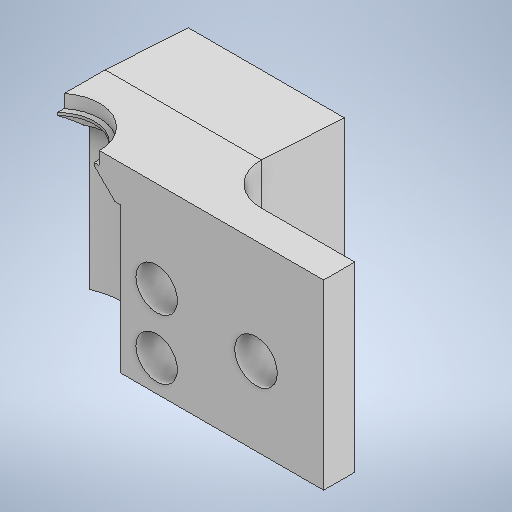
# Autodesk Inventor part: JH_int_Greiferkoerper_Gegenstueck
Saved by Autodesk Inventor 2025.1 (Build 291241000, 241)
## iProperties
Created: 2025-06-16
Part Number: JH_int_Greiferkoerper_Gegenstueck
Material: Generisch
Document SubType Name: Modeling
Designer: Jakob
Density: 1 g/cm^3
Appearance: Vorgabe
Author: Jakob
Autodesk Inventor part; units mm, degrees
ref_plane "YZ Plane" through (0, 0, 0) normal (1, 0, 0) x (0, 1, 0)
ref_plane "XZ Plane" through (0, 0, 0) normal (0, 1, 0) x (-1, 0, 0)
sketch "Skizze1" plane through (0, 0, 0) normal (0, 0, 1) x (1, 0, 0)
  line L0 (6.45, 0) -> (15, 0)
  line L1 (15, 0) -> (15, 15)
  line L2 (15, 15) -> (0, 15)
  line L3 (0, 15) -> (0, 3.0582)
  arc A0 (6.45, 0) -> (0, 3.0582) centre (2.5, 0) ccw
  line L4 (-3, 0) -> (18, 0) projected
  line L5 (0, -3) -> (0, 18) projected
  point P0 (0, 0)
  dimension "d0" = 15
  dimension "d1" = 15
  dimension "d2" = 7.9
  dimension "d3" = 2.5
  constraints: 8 end point, 2 parallel, 2 point on circle, 2 point on line, 1 centre point, 1 collinear, 1 horizontal, 1 perpendicular
  measures "d0" distance of L0.end L1.end
  measures "d1" distance of L1.end L2.end
  measures "d2" diameter of A0
  measures "d3" distance from line of L3 A0.centre
extrude "Extrusion1" add sketch "Skizze1" along normal mid plane 17.5 contours A0 L3 L2 L1 L0
ref_plane "Arbeitsebene1" through (0, 0, 7.5) normal (0, 0, 1) x (1, 0, 0)
sketch "Skizze2" plane through (0, 0, 7.5) normal (0, 0, 1) x (1, 0, 0)
  circle A0 centre (2.5, 0) radius 3.95
  arc A1 (6.45, 0) -> (0, 3.0582) centre (2.5, 0) ccw projected
  circle A2 centre (2.5, 0) radius 3.45
  line L0 (0, 3.0582) -> (0, 2.3775)
  line L1 (15, 0) -> (6.45, 0) projected
  line L2 (6.45, 0) -> (5.95, 0)
  point P0 (0, 0)
  point P1 (0, 3.0582)
  dimension "d7" = 7.9
  dimension "d8" = 6.9
  constraints: 4 end point, 2 centre point, 2 point on circle, 1 coincident, 1 collinear, 1 concentric, 1 vertical
  measures "d7" diameter of A0
  measures "d8" diameter of A2
extrude "Extrusion2" add sketch "Skizze2" against normal up to surface (16.25 mm away) contours L2 A2 L0 A0 picked at (6.25, 0.2945)
sketch "Skizze4" plane through (15, 0, 8.75) normal (1, 0, 0) x (0, 0, -1)
  line L0 (17.5, 3) -> (0, 3)
  line L1 (0, 3) -> (0, 0)
  line L2 (0, 0) -> (17.5, 0)
  line L3 (17.5, 0) -> (17.5, 3)
  line L4 (17.5, 15) -> (17.5, 0) projected
  line L5 (0, 0) -> (0, 15) projected
  line L6 (17.5, 0) -> (0, 0) projected
  point P0 (8.75, 0)
  dimension "d11" = 3
  constraints: 8 end point, 3 collinear, 2 parallel, 1 horizontal, 1 perpendicular
  measures "d11" distance between parallel lines of L2 L0
extrude "Extrusion3" add sketch "Skizze4" along normal blind 13
fillet "Rundung1" radius 4 1 edges at (15, 3, 0)
sketch "Skizze5" plane through (28, 3, 8.75) normal (0, 1, 0) x (1, 0, 0)
  line L0 (-9, 0) -> (0, 0) projected
  line L1 (0, 17.5) -> (0, 0) projected
  point P0 (-28, 8.75)
  point P1 (-6.5, 10)
  dimension "d15" = 10
  dimension "d16" = 6.5
  measures "d15" distance from line of L0 point (-6.5, 10)
  measures "d16" distance from line of L1 point (-6.5, 10)
hole "Bohrung1" at (21.5, 3, -1.25) direction (0, -1, 0) diameter 4.1 end through all
sketch "Skizze6" plane through (5.95, 0, -8.75) normal (0, -1, 0) x (1, 0, 0)
  line L0 (0, 0) -> (22.05, 0) projected
  line L1 (-11.55, 8.75) -> (27.65, 8.75) projected
  line L2 (0, 16.25) -> (0, 0) projected
  point P0 (-5.95, 8.75)
  point P1 (6, 3)
  point P2 (6, 8.75)
  dimension "d24" = 3
  dimension "d25" = 6
  constraints: 1 point on line, 1 vertical alignment
  measures "d24" distance from line of L0 point (6, 3)
  measures "d25" distance from line of L2 point (6, 3)
hole "Bohrung2" at (11.95, 0, -5.75) at (11.95, 0, 0) direction (0, 1, 0) diameter 4 depth 8 tip angle 118
sketch "Skizze7" plane through (0, 0, -8.75) normal (0, 0, -1) x (-1, 0, 0)
  circle A0 centre (-2.5, 0) radius 6
  arc A1 (0, 2.3775) -> (-5.95, 0) centre (-2.5, 0) ccw projected
  line L0 (-5.95, 0) -> (-8.5, 0)
  line L1 (-5.95, 0) -> (-28, 0) projected
  line L2 (0, 2.3775) -> (0, 15) projected
  line L3 (0, 2.3775) -> (0, 5.4544)
  point P0 (0, 0)
  dimension "d34" = 12
  constraints: 4 end point, 2 point on circle, 2 point on line, 1 centre point, 1 concentric
  measures "d34" diameter of A0
extrude "Extrusion4" cut sketch "Skizze7" against normal blind 14 contours L2 A1 L0 A0 picked at (-7.6008, 0.4409)
chamfer "Fasen1" distance 2 angle 45 1 edges at (3.7801, 3.2037, 5.25)
sketch "Skizze8" plane through (0, 3.0582, 8.75) normal (-1, 0, 0) x (0, 0, 1)
  line L0 (0, 3.9418) -> (0, 11.9418) projected
  line L1 (0, 3.9418) -> (-0.5, 11.9418)
  line L2 (-17.5, 11.9418) -> (0, 11.9418) projected
  line L3 (-0.5, 11.9418) -> (0, 11.9418)
  line L4 (0, 11.9418) -> (0, 3.9418)
  point P0 (-8.75, -3.0582)
  dimension "d40" = 8
  dimension "d41" = 0.5
  constraints: 6 end point, 1 collinear, 1 perpendicular, 1 point on line
  measures "d40" distance from line of L0.start L2
  measures "d41" distance from line of L0 L1.end
extrude "Extrusion5" cut sketch "Skizze8" against normal through all
equation "\"d0\" = Tiefe_Gegenstueck"
equation "\"d1\" = Breite_Grundkoerper"
equation "\"d2\" = D_Scheibe"
equation "\"d3\" = Abstand_D_Scheibe"
equation "\"d4\" = Tiefe_Grundkoerper"
equation "\"d7\" = D_Scheibe"
equation "\"d11\" = Breite_Absatz"
equation "\"d12\" = Tiefe_Absatz"
equation "\"d14\" = Radius_Absatz"
equation "\"d15\" = Pos_Bohrung_Kolben_y"
equation "\"d16\" = Pos_Bohrung_Kolben_x"
equation "\"d17\" = D_Kolbenbohrung"
equation "\"d24\" = Zentrierbohrung_y"
equation "\"d25\" = Zentrierbohrung_x"
equation "\"d26\" = D_Zentrierbohrung"
equation "\"d31\" = T_Zentrierbohrung"
equation "\"Breite_Grundkoerper\" = 15"
equation "\"D_Scheibe\" = 7.9"
equation "\"Abstand_D_Scheibe\" = 2.5"
equation "\"Abstand_Arbeitsebene\" = 2"
equation "\"Tiefe_Grundkoerper\" = 17.5"
equation "\"Tiefe_Gegenstueck\" = 15"
equation "\"Breite_Absatz\" = 3"
equation "\"Tiefe_Absatz\" = 13"
equation "\"Radius_Absatz\" = 4"
equation "\"Pos_Bohrung_Kolben_x\" = 6.5"
equation "\"Pos_Bohrung_Kolben_y\" = 10"
equation "\"D_Kolbenbohrung\" = 4.1"
equation "\"Zentrierbohrung_y\" = 3"
equation "\"T_Zentrierbohrung\" = 8"
equation "\"D_Zentrierbohrung\" = 4"
equation "\"Zentrierbohrung_x\" = 6"
equation "\"R_Kanten\" = 0.5"
